9c0b87b4-3cfa-454a-bccc-b9391833bb94 (Autodesk Fusion 360 design; units mm, degrees)
Autodesk Fusion 360 part; units mm, degrees
sketch "Sketch1" plane through (0, 0, 0) normal (0, 1, 0) x (1, 0, 0)
  circle A0 centre (0, 0) radius 10.5791
  circle A1 centre (0, 0) radius 11.684
  circle A2 centre (0, 0) radius 9.5212
  circle A3 centre (0, 0) radius 9.9411
  arc A4 (11.6541, -0.8359) -> (-10.7093, -4.672) centre (0, 0) ccw
  circle A5 centre (0, 0) radius 0.3969
  line L0 (0, 0) -> (11.684, 0) construction
  line L1 (0, 0) -> (-0.8664, -9.9033)
  line L2 (0, 0) -> (-1.7263, -9.7901)
  line L3 (0, 0) -> (-2.5729, -9.6024)
  line L4 (0, 0) -> (-3.4001, -9.3416)
  line L5 (0, 0) -> (-4.2013, -9.0097)
  line L6 (0, 0) -> (-4.9706, -8.6092)
  line L7 (0, 0) -> (-5.702, -8.1433)
  line L8 (-0.8664, -9.9033) -> (-0.0022, -9.9789) construction
  line L9 (-1.7263, -9.7901) -> (-0.0176, -10.0914) construction
  line L10 (-2.5729, -9.6024) -> (-0.0591, -10.276) construction
  line L11 (-3.4001, -9.3416) -> (-0.1392, -10.5284) construction
  line L12 (-4.2013, -9.0097) -> (-0.2701, -10.8429) construction
  line L13 (-4.9706, -8.6092) -> (-0.4628, -11.2118) construction
  line L14 (-5.702, -8.1433) -> (-0.7275, -11.6264) construction
  line L15 (0, 0) -> (-6.39, -7.6153)
  line L16 (-6.39, -7.6153) -> (-1.0735, -12.0764) construction
  line L17 (0, 0) -> (-7.0294, -7.0294)
  line L18 (-7.0294, -7.0294) -> (-1.5085, -12.5503) construction
  spline S0 degree 5 poles (-1.5085, -12.5503) (-1.495, -12.5338) (-1.4678, -12.501) (-1.4264, -12.4528) (-1.3702, -12.3904) (-1.2991, -12.3149) (-1.228, -12.2411) (-1.1578, -12.1681) (-1.0896, -12.0951) (-1.0241, -12.0215) (-0.9617, -11.9469) (-0.9023, -11.8715) (-0.8456, -11.7956) (-0.7913, -11.7195) (-0.7391, -11.6438) (-0.6884, -11.5687) (-0.6393, -11.4945) (-0.5917, -11.4213) (-0.5457, -11.3489) (-0.5015, -11.2774) (-0.4592, -11.2065) (-0.4191, -11.1363) (-0.3812, -11.0668) (-0.3453, -10.9981) (-0.3114, -10.9304) (-0.2795, -10.8637) (-0.2494, -10.7983) (-0.2211, -10.7343) (-0.1947, -10.6717) (-0.1701, -10.6107) (-0.1473, -10.5512) (-0.1264, -10.4934) (-0.1073, -10.4374) (-0.09, -10.3833) (-0.0744, -10.3314) (-0.0604, -10.2818) (-0.048, -10.2346) (-0.0372, -10.1901) (-0.028, -10.1482) (-0.0204, -10.1091) (-0.0144, -10.0731) (-0.0097, -10.0405) (-0.0061, -10.0118) (-0.0032, -9.9875) (-0.0009, -9.968) (0.0007, -9.9536) (0.0011, -9.9461) (0.0008, -9.9427) (0.0003, -9.9415) (0, -9.9411) knots 0 0 0 0 0 0 0.022222 0.044444 0.066667 0.088889 0.111111 0.133333 0.155556 0.177778 0.2 0.222222 0.244444 0.266667 0.288889 0.311111 0.333333 0.355556 0.377778 0.4 0.422222 0.444444 0.466667 0.488889 0.511111 0.533333 0.555556 0.577778 0.6 0.622222 0.644444 0.666667 0.688889 0.711111 0.733333 0.755556 0.777778 0.8 0.822222 0.844444 0.866667 0.888889 0.911111 0.933333 0.955556 0.977778 1 1 1 1 1 1
  line L19 (-1.6062, -12.6699) -> (-1.4108, -12.4307)
  line L20 (0.0201, -9.964) -> (-0.0201, -9.9182)
  line L21 (-0.1577, -10.5779) -> (0, 0)
  line L22 (0, 0) -> (-0.5708, -6.0907) construction
  line L23 (0, -9.9411) -> (0, 0) construction
  spline S1 degree 5 poles (0, -9.9411) (0, -9.9159) (0, -9.8689) (0, -9.8083) (0, -9.7442) (0, -9.6772) (0, -9.6223) (0, -9.5749) (0, -9.5397) (0, -9.5212) knots 0 0 0 0 0 0 0.2 0.4 0.6 0.8 1 1 1 1 1 1
  spline S2 degree 5 poles (-1.8471, -9.768) (-1.8425, -9.7432) (-1.8337, -9.697) (-1.8225, -9.6375) (-1.8106, -9.5745) (-1.7981, -9.5087) (-1.7879, -9.4548) (-1.7791, -9.4082) (-1.7726, -9.3736) (-1.7691, -9.3554) knots 0 0 0 0 0 0 0.2 0.4 0.6 0.8 1 1 1 1 1 1
  line L24 (0, -10.0186) -> (0, -9.8636)
  line L25 (0, -9.5782) -> (0, -9.4642)
  line L26 (-1.8615, -9.8442) -> (-1.8327, -9.6918)
  line L27 (-1.7797, -9.4114) -> (-1.7585, -9.2994)
  spline S3 degree 5 poles (-0.8497, -12.6121) (-0.8599, -12.5933) (-0.8806, -12.556) (-0.9123, -12.5009) (-0.9559, -12.4292) (-1.0117, -12.3418) (-1.0679, -12.2561) (-1.1233, -12.1714) (-1.1767, -12.087) (-1.2274, -12.0024) (-1.2749, -11.9175) (-1.3193, -11.8324) (-1.3608, -11.7473) (-1.4, -11.6625) (-1.4373, -11.5783) (-1.4731, -11.4952) (-1.5076, -11.4132) (-1.5408, -11.3323) (-1.5726, -11.2527) (-1.6027, -11.1742) (-1.631, -11.0967) (-1.6574, -11.0203) (-1.6818, -10.9449) (-1.7043, -10.8708) (-1.725, -10.7979) (-1.7439, -10.7265) (-1.7614, -10.6566) (-1.7772, -10.5885) (-1.7916, -10.5221) (-1.8045, -10.4575) (-1.8158, -10.3948) (-1.8256, -10.3341) (-1.8339, -10.2755) (-1.8408, -10.2192) (-1.8465, -10.1653) (-1.8511, -10.114) (-1.8545, -10.0653) (-1.8569, -10.0195) (-1.8581, -9.9767) (-1.8583, -9.9369) (-1.8575, -9.9003) (-1.856, -9.8674) (-1.8543, -9.8386) (-1.8526, -9.8142) (-1.8513, -9.7946) (-1.8502, -9.7801) (-1.8492, -9.7727) (-1.8483, -9.7694) (-1.8475, -9.7683) (-1.8471, -9.768) knots 0 0 0 0 0 0 0.022222 0.044444 0.066667 0.088889 0.111111 0.133333 0.155556 0.177778 0.2 0.222222 0.244444 0.266667 0.288889 0.311111 0.333333 0.355556 0.377778 0.4 0.422222 0.444444 0.466667 0.488889 0.511111 0.533333 0.555556 0.577778 0.6 0.622222 0.644444 0.666667 0.688889 0.711111 0.733333 0.755556 0.777778 0.8 0.822222 0.844444 0.866667 0.888889 0.911111 0.933333 0.955556 0.977778 1 1 1 1 1 1
  line L28 (-0.7759, -12.7478) -> (-0.9235, -12.4764)
  line L29 (-1.8712, -9.7868) -> (-1.8231, -9.7492)
  point P0 (-0.1577, -10.5779)
  point P1 (0, -9.5212)
  point P2 (-1.1891, -12.0656)
  point P3 (-1.4454, -11.5591)
  point P4 (-1.6285, -11.1026)
  point P5 (-1.7493, -10.7042)
  point P6 (-1.8195, -10.371)
  point P7 (-1.8513, -10.108)
  point P8 (-1.8578, -9.9189)
  point P9 (-1.852, -9.8055)
  point P10 (-1.7691, -9.3554)
  dimension "d2" = 23.368
  dimension "id" = 19.0424
  dimension "BaseDiameter" = 19.8822
  dimension "d1" = 0.7937
  dimension "d34" = 5
  dimension "d35" = 5
  dimension "d36" = 5
  dimension "d37" = 5
  dimension "d38" = 5
  dimension "d39" = 5
  dimension "d41" = 0.8675
  dimension "d42" = 1.735
  dimension "d43" = 2.6026
  dimension "d44" = 3.4701
  dimension "d45" = 4.3376
  dimension "d46" = 5.2051
  dimension "d47" = 6.0727
  dimension "d48" = 5
  dimension "d49" = 6.9402
  dimension "d50" = 5
  dimension "d51" = 7.8077
  dimension "d55" = 4.5
  dimension "d60" = 5
  constraint coincident A0.centre A1.centre
  constraint concentric A0 A2
  constraint coincident A1 A4.end
  constraint horizontal L0
  constraint coincident A4 L0.end
  constraint coincident A3 S0.end
  constraint coincident A3 L1.end
  constraint coincident A3 L2.end
  constraint coincident A3 L3.end
  constraint coincident A3 L4.end
  constraint coincident A3 L5.end
  constraint coincident A3 L6.end
  constraint coincident A3 L7.end
  constraint vertical A0.centre S0.end
  constraint tangent A3 L8
  constraint tangent A3 L9
  constraint tangent A3 L10
  constraint tangent A3 L11
  constraint tangent A3 L12
  constraint tangent A3 L13
  constraint tangent A3 L14
  constraint coincident A3 L15.end
  constraint tangent A3 L16
  constraint coincident A3 L17.end
  constraint tangent A3 L18
  constraint midpoint L18.end L19
  constraint midpoint S0.end L20
  constraint coincident A0 P0
  constraint coincident S0 P0
  constraint coincident P0 L21.start
  constraint coincident L23 P1
  constraint coincident A2 P1
  constraint coincident P1 S1.end
  constraint midpoint S0.end L24
  constraint midpoint P1 L25
  constraint symmetric S0.end L22 S2.start
  constraint symmetric L8.end L22 P9
  constraint symmetric L9.end L22 P8
  constraint symmetric L10.end L22 P7
  constraint symmetric L11.end L22 P6
  constraint symmetric L12.end L22 P5
  constraint symmetric L13.end L22 P4
  constraint symmetric L14.end L22 P3
  constraint symmetric L16.end L22 P2
  constraint symmetric L18.end L22 S3.start
  constraint symmetric L19.start L22 L28.start
  constraint symmetric L19.end L22 L28.end
  constraint symmetric L20.start L22 L29.start
  constraint symmetric L20.end L22 L29.end
  constraint symmetric L22 P1 P10
  constraint symmetric L22 L24.start L26.start
  constraint symmetric L22 L24.end L26.end
  constraint symmetric L22 L25.start L27.start
  constraint symmetric L22 L25.end L27.end
  constraint vertical L24
  constraint vertical L25
  measures "d2" diameter of A1
  measures "id" diameter of A2
  measures "BaseDiameter" diameter of A3
  measures "d1" diameter of A5
  measures "d34" angle of L1 L2
  measures "d35" angle of L2 L3
  measures "d36" angle of L3 L4
  measures "d37" angle of L4 L5
  measures "d38" angle of L5 L6
  measures "d39" angle of L6 L7
  measures "d41" distance of L1.end L8.end
  measures "d42" distance of L2.end L9.end
  measures "d43" distance of L3.end L10.end
  measures "d44" distance of L4.end L11.end
  measures "d45" distance of L5.end L12.end
  measures "d46" distance of L6.end L13.end
  measures "d47" distance of L7.end L14.end
  measures "d48" angle of L7 L15
  measures "d49" distance of L15.end L16.end
  measures "d50" angle of L15 L17
  measures "d51" distance of L17.end L18.end
  measures "d55" angle of L21 L22
  measures "d60" angle of L1 L23
extrude "Extrude1" add sketch "Sketch1" along normal blind 304.8 contours A0 A1 S0 S3 | A3 S0 L21 | A0 A3 L21 S3 | A2 A3 L21 S1 L24 L25 | A2 A3 L1 L21 | A2 A3 L2 S2 L26 L27 | A2 A3 L1 L2 makes body 1
pattern_circular "C-Pattern2" count 12 over 360 about axis through (0, 1.75, 0) along (0, 1, 0) of bodies 1 makes body 2 at (3.8804, 203.2, 8.6946) makes body 3 at (7.7078, 203.2, 5.5896) makes body 4 at (9.4699, 203.2, 0.9868) makes body 5 at (8.6946, 203.2, -3.8804) makes body 6 at (5.5896, 203.2, -7.7078) makes body 7 at (0.9868, 203.2, -9.4699) makes body 8 at (-3.8804, 203.2, -8.6946) makes body 9 at (-7.7078, 203.2, -5.5896) makes body 10 at (-9.4699, 203.2, -0.9868) makes body 11 at (-8.6946, 203.2, 3.8804) makes body 12 at (-5.5896, 203.2, 7.7078)
extrude "Extrude2" add sketch "Sketch1" along normal blind 304.8 contours A2 A5 L17 L21 | A2 A5 L1 L21 | A2 A5 L1 L2 | A2 A5 L2 L3 | A2 A5 L3 L4 | A2 A5 L15 L17 | A2 A5 L4 L5 | A2 A5 L7 L15 | A2 A5 L5 L6 | A2 A5 L6 L7 bodies 1 2 3 4 5 6 7 8 9 10 11 12
ref_plane "WorkPlane1" through (6.2747, 152.4, -0.8261) normal (0.130526, 0, 0.991445) x (0.991445, 0, -0.130526)
fillet "Fillet1" [suppressed]
mirror "Mirror3" [suppressed]
pattern_circular "C-Pattern1" [suppressed]
equation "d = 0.833 in"
equation "OutsideDiameter = d2"
equation "PitchDiameter = d"
equation "id = PitchDiameter - 2 * ( PitchDiameter / TeethNumber )"
equation "BaseDiameter = PitchDiameter * cos(20 deg)"
equation "Length = 12 in"
equation "t = 20"
equation "ShaftDiameter = d1"
equation "TeethNumber = t"
equation "Pitch = 32"
equation "d30 = ( 1.25 * ( PitchDiameter / TeethNumber ) ) - ( PitchDiameter / TeethNumber )"
equation "Basecircum = PI * PitchDiameter * cos(20 deg)"
equation "d41 = Basecircum * 5 / 360"
equation "d42 = Basecircum * 10 / 360"
equation "d43 = Basecircum * 15 / 360"
equation "d44 = Basecircum * 20 / 360"
equation "d45 = Basecircum * 25 / 360"
equation "d46 = Basecircum * 30 / 360"
equation "d47 = Basecircum * 35 / 360"
equation "d49 = Basecircum * 40 / 360"
equation "d51 = Basecircum * 45 / 360"
equation "d55 = ( 360 / ( 4 * TeethNumber ) ) * 1 deg"
